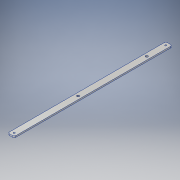
# Autodesk Inventor part: Compressor_Strut
Saved by Autodesk Inventor 2016 (Build 200138000, 138)
## iProperties
Created: 2016-03-26
Part Number: Compressor_Strut
Material: Aluminum 6061
Document SubType Name: Sheet Metal
Designer: agmle
Density: 2.7 g/cm^3
Sheet Metal Rule: Default
Appearance: Aluminum - Flat
Author: agmle
Autodesk Inventor part; units mm, degrees
ref_plane "YZ Plane" through (0, 0, 0) normal (1, 0, 0) x (0, 1, 0)
ref_plane "XZ Plane" through (0, 0, 0) normal (0, 1, 0) x (-1, 0, 0)
ref_plane "XY Plane" through (0, 0, 0) normal (0, 0, 1) x (1, 0, 0)
sketch "Sketch1" plane through (0, 0, 0) normal (0, 1, 0) x (-1, 0, 0)
  line L0 (8.5925, 12.671) -> (-4.1075, 12.671)
  line L1 (-4.1075, 12.671) -> (-4.1075, -304.829)
  line L2 (-4.1075, -304.829) -> (8.5925, -304.829)
  line L3 (8.5925, -304.829) -> (8.5925, 12.671)
  point P0 (0, 0)
  dimension "d0" = 12.7
  dimension "d1" = 317.5
  measures "d0" distance of L0.start L0.end
  measures "d1" distance of L2.end L0.start
extrude "Plate1" add sketch "Sketch1" along normal blind 3.048
fillet "Corner Round1" radius 3.175 4 edges at (4.1075, 1.524, 12.671) (-8.5925, 1.524, 12.671) (-8.5925, 1.524, -304.829) (4.1075, 1.524, -304.829)
sketch "Sketch2" plane through (0, 3.048, 0) normal (0, 1, 0) x (1, 0, 0)
  line L0 (0.9325, -12.671) -> (-5.4175, -12.671) projected
  line L1 (4.1075, 301.654) -> (4.1075, -9.496) projected
  line L2 (-5.4175, 304.829) -> (0.9325, 304.829) projected
  point P0 (0, 0)
  point P1 (-2.2425, -6.321)
  point P2 (-2.2425, 298.479)
  dimension "d4" = 6.35
  dimension "d5" = 6.35
  dimension "d6" = 6.35
  dimension "d7" = 6.35
  measures "d4" distance from line of L0 point (-2.242, -6.321)
  measures "d5" distance from line of L1 point (-2.242, -6.321)
  measures "d6" distance from line of L2 point (-2.242, 298.479)
  measures "d7" distance from line of L1 point (-2.242, 298.479)
hole "Hole1" at (-2.2425, 3.048, 6.321) at (-2.2425, 3.048, -298.479) direction (0, -1, 0) diameter 3.2766 end through all clearance for "Flat Head Machine Screw (82)" size "#4" standard "Ansi Unified Screw Threads"
sketch "Sketch3" plane through (0, 3.048, 0) normal (0, 1, 0) x (1, 0, 0)
  line L0 (4.1075, 301.654) -> (4.1075, -9.496) projected
  circle A0 centre (-2.2425, 298.479) radius 1.6383 projected
  point P0 (0, 0)
  point P1 (-2.2425, 260.379)
  point P2 (-2.2425, 122.2284)
  dimension "d15" = 6.35
  dimension "d16" = 6.35
  dimension "d17" = 138.1506
  dimension "d18" = 38.1
  measures "d15" distance from line of L0 point (-2.242, 260.379)
  measures "d16" distance from line of L0 point (-2.242, 122.228)
  measures "d17" distance of point (-2.242, 122.228) point (-2.242, 260.379)
  measures "d18" distance of A0.centre point (-2.242, 260.379)
hole "Hole2" at (-2.2425, 3.048, -260.379) at (-2.2425, 3.048, -122.2284) direction (0, -1, 0) diameter 4.9784 end through all thread size "1/4-20 UNC" class "2B" standard "ANSI Unified Screw Threads"
equation "\"BendRadius\" = Thickness"
equation "\"BendReliefWidth\" = Thickness"
equation "\"BendReliefDepth\" = 0.5 * Thickness"
equation "\"CornerReliefSize\" = 4 * Thickness"
equation "\"MinimumRemnant\" = 2 * Thickness"
equation "\"TransitionRadius\" = BendRadius"
equation "\"JacobiRadiusSize\" = BendRadius"
equation "\"GapSize\" = Thickness"
equation "\"d2\" = BendRadius"
equation "\"Thickness\" = 3.048"
body "Solid1"
